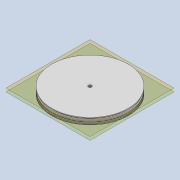
# Autodesk Inventor part: roller_2
Saved by Autodesk Inventor 2020 (Build 240168000, 168)
## iProperties
Created: 2021-09-11
Part Number: roller_2
Material: Generic
Document SubType Name: Modeling
Designer: Shuang Peng
Density: 1 g/cm^3
Appearance: Default
Author: Shuang Peng
Autodesk Inventor part; units mm, degrees
ref_plane "YZ Plane" through (0, 0, 0) normal (1, 0, 0) x (0, 1, 0)
ref_plane "XZ Plane" through (0, 0, 0) normal (0, 1, 0) x (-1, 0, 0)
ref_plane "XY Plane" through (0, 0, 0) normal (0, 0, 1) x (1, 0, 0)
sketch "Sketch1" plane through (0, 0, 0) normal (0, 1, 0) x (-1, 0, 0)
  circle A0 centre (0, 0) radius 35
  dimension "d0" = 70
  constraints: 1 centre point, 1 coincident
  measures "d0" diameter of A0
extrude "Extrusion1" add sketch "Sketch1" along normal blind 6
ref_plane "Work Plane1" through (0, 4.5, 0) normal (0, 1, 0) x (1, 0, 0)
ref_plane "Work Plane2" through (0, 1.5, 0) normal (0, -1, 0) x (1, 0, 0)
sketch "Sketch2" plane through (0, 6, 0) normal (0, 1, 0) x (1, 0, 0)
  circle A0 centre (0, 0) radius 1.5
  dimension "d5" = 3
  constraints: 1 centre point, 1 coincident
  measures "d5" diameter of A0
extrude "Extrusion2" cut sketch "Sketch2" against normal blind 6
sketch "Sketch3" plane through (0, 0, 0) normal (1, 0, 0) x (0, 1, 0)
  line L0 (0, 35) -> (6, 35) projected
  line L1 (6, 35) -> (4.4, 35)
  line L2 (4.4, 35) -> (4.4, 34.5)
  line L3 (5.4, 33.5) -> (5.4, 35.5)
  line L4 (5.4, 35.5) -> (3.4, 35.5)
  line L5 (3.4, 35.5) -> (3.4, 33.5)
  line L6 (3.4, 33.5) -> (5.4, 33.5)
  line L7 (5.4, 33.5) -> (3.4, 35.5) construction
  line L8 (5.4, 35.5) -> (3.4, 33.5) construction
  line L9 (0, -35) -> (0, 35) projected
  line L10 (0, 35) -> (1.6, 35)
  line L11 (1.6, 35) -> (1.6, 34.5)
  line L12 (2.6, 33.5) -> (2.6, 35.5)
  line L13 (2.6, 35.5) -> (0.6, 35.5)
  line L14 (0.6, 35.5) -> (0.6, 33.5)
  line L15 (0.6, 33.5) -> (2.6, 33.5)
  line L16 (2.6, 33.5) -> (0.6, 35.5) construction
  line L17 (2.6, 35.5) -> (0.6, 33.5) construction
  line L18 (0, 0) -> (10, 0)
  point P0 (2.6, 35)
  point P1 (0.6, 35)
  point P2 (5.4, 35)
  point P3 (3.4, 35)
  dimension "d8" = 1.6
  dimension "d9" = 0.5
  dimension "d10" = 2
  dimension "d11" = 2
  dimension "d12" = 1.6
  dimension "d13" = 0.5
  dimension "d14" = 2
  dimension "d15" = 2
  dimension "d16" = 10
  constraints: 34 end point, 5 parallel, 4 midpoint, 3 perpendicular, 2 point on line, 2 vertical, 1 horizontal
  measures "d8" distance of L0.end L1.end
  measures "d9" distance of L1.end L2.end
  measures "d10" distance of L3.start L3.end
  measures "d11" distance of L4.end L3.end
  measures "d12" distance of L0.start L10.end
  measures "d13" distance of L10.end L11.end
  measures "d14" distance of L12.start L12.end
  measures "d15" distance of L13.end L12.end
  measures "d16" distance of L18.start L18.end
revolve "Revolution1" cut sketch "Sketch3" angle 360 about axis through (0, 0, 0) along (0, 1, 0) contours L0 L3 L6 L5 | L0 L12 L15 L14
fillet "Fillet1" radius 0.5 4 edges at (0, 3.4, -33.5) (0, 5.4, -33.5) (0, 2.6, -33.5) (0, 0.6, -33.5)
body "Solid1"
